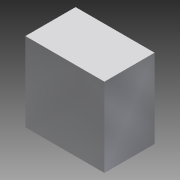
# Autodesk Inventor part: ColdFingerBase
Saved by Autodesk Inventor 2014 (Build 180170000, 170)
## iProperties
Created: 2015-04-18
Part Number: ColdFingerBase
Material: Generic
Document SubType Name: Modeling
Designer: Owner
Density: 1 g/cm^3
Appearance: Aluminum - Polished
Author: Owner
Autodesk Inventor part; units mm, degrees
ref_plane "YZ Plane" through (0, 0, 0) normal (1, 0, 0) x (0, 1, 0)
ref_plane "XZ Plane" through (0, 0, 0) normal (0, 1, 0) x (-1, 0, 0)
ref_plane "XY Plane" through (0, 0, 0) normal (0, 0, 1) x (1, 0, 0)
sketch "Sketch2" plane through (0, 0, 0) normal (0, 0, 1) x (1, 0, 0)
  line L0 (-19.5826, 20.0613) -> (20.4174, 20.0613)
  line L1 (20.4174, 20.0613) -> (20.4174, -19.9387)
  line L2 (20.4174, -19.9387) -> (-19.5826, -19.9387)
  line L3 (-19.5826, -19.9387) -> (-19.5826, 20.0613)
  point P0 (0, 0)
  dimension "d0" = 40
  dimension "d1" = 40
  constraints: 8 end point, 2 parallel, 1 horizontal, 1 perpendicular
  measures "d0" distance of L0.start L0.end
  measures "d1" distance of L0.end L1.end
extrude "Extrusion1" add sketch "Sketch2" along normal blind 6.35
sketch "Sketch3" plane through (0, 0, 6.35) normal (0, 0, 1) x (1, 0, 0)
  line L0 (20.4174, 20.0613) -> (-19.5826, 20.0613) projected
  line L1 (20.4174, -19.9387) -> (20.4174, 20.0613) projected
  line L2 (-9.5826, 10.0613) -> (10.4174, 10.0613)
  line L3 (10.4174, 10.0613) -> (10.4174, -9.9387)
  line L4 (10.4174, -9.9387) -> (-9.5826, -9.9387)
  line L5 (-9.5826, -9.9387) -> (-9.5826, 10.0613)
  point P0 (0, 0)
  dimension "d4" = 20
  dimension "d5" = 20
  dimension "d6" = 10
  dimension "d7" = 10
  constraints: 8 end point, 2 parallel, 1 horizontal, 1 perpendicular
  measures "d4" distance of L2.start L2.end
  measures "d5" distance of L2.end L3.end
  measures "d6" distance between parallel lines of L0 L2
  measures "d7" distance between parallel lines of L1 L3
extrude "Extrusion2" add sketch "Sketch3" along normal blind 20
body "Solid1"
